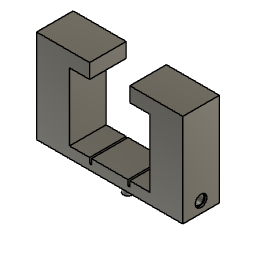
MotorHolder v1 (MostComplicated) (Autodesk Fusion 360 design; units mm, degrees)
Autodesk Fusion 360 part; units mm, degrees
sketch "Sketch1" plane through (0, 0, 0) normal (0, 0, 1) x (1, 0, 0)
  line L0 (25, -9.25) -> (-25, -9.25)
  line L1 (-25, -9.25) -> (-25, 9.25)
  line L2 (-25, 9.25) -> (25, 9.25)
  line L3 (25, 9.25) -> (25, -9.25)
  line L4 (25, -9.25) -> (-25, 9.25) construction
  line L5 (-25, -9.25) -> (25, 9.25) construction
  dimension "d1" = 50
  dimension "d2" = 18.5
  constraint horizontal L0
  constraint perpendicular L0 L1
  constraint parallel L0 L2
  constraint parallel L1 L3
  constraint coincident L4 origin
  constraint coincident L5 origin
  measures "d1" distance of L1.end L2.end
  measures "d2" distance of L0.end L1.end
extrude "Extrude1" add sketch "Sketch1" along normal blind 22 makes body 1
move_body "Move1" bodies 1 to x (0, -1, 0) y (1, 0, 0) z (0, 0, 1) at (9.25, -34.25, 0)
move_body "Move2" bodies 1 to x (1, 0, 0) y (0, 1, 0) z (0, 0, 1) at (0, 34, 0)
sketch "Sketch2" plane through (0, 0, 0) normal (0, 0, 1) x (1, 0, 0)
  line L0 (20, 6) -> (30, 6)
  line L1 (30, 6) -> (30, -8.5)
  line L2 (30, -8.5) -> (20, -8.5)
  line L3 (20, -8.5) -> (20, 6)
  dimension "d5" = 10
  dimension "d6" = 14.5
  constraint horizontal L0
  constraint vertical L1
  constraint horizontal L2
  constraint vertical L3
  measures "d5" distance of L0.start L0.end
  measures "d6" distance of L0.start L2.end
extrude "Extrude2" add sketch "Sketch2" along normal blind 24 separate body makes body 2
move_body "Move3" bodies 1 to x (0, 0, 1) y (0, 1, 0) z (-1, 0, 0) at (11, 0, 0)
move_body "Move4" bodies 2 to x (1, 0, 0) y (0, 1, 0) z (0, 0, 1) at (-9, 0, 0)
move_body "Move5" bodies 2 to x (0, -1, 0) y (1, 0, 0) z (0, 0, 1) at (19.5, 2.5, 0)
move_body "Move6" bodies 2 to x (1, 0, 0) y (0, 1, 0) z (0, 0, 1) at (0, 14, 0)
copy_body "CopyPasteBodies1" bodies 2 makes body 3
move_body "Move7" bodies 3 to x (1, 0, 0) y (0, 1, 0) z (0, 0, 1) at (-37, 0, 0)
sketch "Sketch3" plane through (0, 0, 0) normal (0, 0, 1) x (1, 0, 0)
  line L0 (-6, 4) -> (4, 4)
  line L1 (4, 4) -> (4, -6)
  line L2 (4, -6) -> (-6, -6)
  line L3 (-6, -6) -> (-6, 4)
  dimension "d9" = 10
  dimension "d10" = 10
  constraint horizontal L0
  constraint vertical L1
  constraint horizontal L2
  constraint vertical L3
  measures "d9" distance of L0.start L0.end
  measures "d10" distance of L0.start L2.end
extrude "Extrude3" add sketch "Sketch3" along normal blind 3 separate body makes body 4
move_body "Move8" bodies 4 to x (1, 0, 0) y (0, 1, 0) z (0, 0, 1) at (0, 0, -3)
move_body "Move9" bodies 4 to x (1, 0, 0) y (0, 1, 0) z (0, 0, 1) at (1, 1, 0)
move_body "Move10" bodies 2 3 to x (1, 0, 0) y (0, 1, 0) z (0, 0, 1) at (0, 0, -1.5)
move_body "Move11" bodies 2 to x (1, 0, 0) y (0, 1, 0) z (0, 0, 1) at (-6, 0, 0)
move_body "Move12" bodies 3 to x (1, 0, 0) y (0, 1, 0) z (0, 0, 1) at (6, 0, 0)
move_body "Move13" bodies 3 to x (1, 0, 0) y (0, 1, 0) z (0, 0, 1) at (0.5, 0, 0)
sketch "Sketch4" plane through (0, 0, 18.5) normal (0, 0, 1) x (-1, 0, 0)
  line L0 (-11, 25.25) -> (-11, -24.75)
  line L1 (-11, -24.75) -> (11, -24.75)
  line L2 (11, -24.75) -> (11, 25.25)
  line L3 (11, 25.25) -> (-11, 25.25)
  line L4 (-20, 5) -> (20, 5)
  line L5 (20, 5) -> (20, -5)
  line L6 (20, -5) -> (-20, -5)
  line L7 (-20, -5) -> (-20, 5)
  line L8 (-20, 5) -> (20, -5) construction
  line L9 (20, 5) -> (-20, -5) construction
  dimension "d13" = 40
  dimension "d14" = 10
  constraint horizontal L4
  constraint perpendicular L4 L5
  constraint parallel L4 L6
  constraint parallel L5 L7
  constraint coincident L8 origin
  constraint coincident L9 origin
  measures "d13" distance of L5.end L6.end
  measures "d14" distance of L4.end L5.end
extrude "Extrude4" add sketch "Sketch4" along normal blind 1.5 separate body contours L0 L2 L4 L6 | L0 L4 L6 L7 | L2 L4 L5 L6 makes body 5
move_body "Move14" bodies 5 to x (1, 0, 0) y (0, 1, 0) z (0, 0, 1) at (0, 0, -21.5)
move_body "Move15" bodies 3 to x (1, 0, 0) y (0, 1, 0) z (0, 0, 1) at (-0.5, 0, 0)
move_body "Move16" bodies 2 to x (1, 0, 0) y (0, 1, 0) z (0, 0, 1) at (0.5, 0, 0)
sketch "Sketch5" plane through (0, 0, 0) normal (0, 0, 1) x (1, 0, 0)
  circle A0 centre (0, 0) radius 1.255
  dimension "d17" = 2.51
  constraint coincident A0.centre origin
  measures "d17" diameter of A0
extrude "Extrude5" add sketch "Sketch5" against normal blind 8 bodies 4 5
sketch "Sketch6" plane through (0, 0, -3) normal (0, 0, -1) x (1, 0, 0)
  circle A0 centre (0, 0) radius 1.255
  line L0 (20, 5) -> (-20, 5)
  line L1 (-20, 5) -> (-20, -5)
  line L2 (-20, -5) -> (20, -5)
  line L3 (20, -5) -> (20, 5)
  circle A1 centre (0, 0) radius 1.6
  dimension "d20" = 3.2
  constraint concentric A0 A1
  measures "d20" diameter of A1
extrude "Extrude6" add sketch "Sketch6" along normal blind 0.5 contours A1 bodies 4
sketch "Sketch7" plane through (20, 0, 0) normal (1, 0, 0) x (0, 1, 0)
  line L0 (-4.5, -1.5) -> (5.5, -1.5)
  line L1 (5.5, -1.5) -> (5.5, 22.5)
  line L2 (5.5, 22.5) -> (-4.5, 22.5)
  line L3 (-4.5, 22.5) -> (-4.5, -1.5)
  circle A0 centre (0, 0) radius 1.3
  dimension "d23" = 2.6
  constraint coincident A0.centre origin
  measures "d23" diameter of A0
move_body "Move18" bodies 2 to x (1, 0, 0) y (0, 1, 0) z (0, 0, 1) at (0, -0.5, 0)
move_body "Move19" bodies 3 to x (1, 0, 0) y (0, 1, 0) z (0, 0, 1) at (0, -0.5, 0)
sketch "Sketch9" plane through (20, 0, 0) normal (1, 0, 0) x (0, 1, 0)
  line L0 (-5, -1.5) -> (5, -1.5)
  line L1 (5, -1.5) -> (5, 22.5)
  line L2 (5, 22.5) -> (-5, 22.5)
  line L3 (-5, 22.5) -> (-5, -1.5)
  circle A0 centre (0, 0) radius 1.3
  dimension "d29" = 2.6
  constraint coincident A0.centre origin
  measures "d29" diameter of A0
extrude "Extrude9" cut sketch "Sketch9" against normal blind 8 contours A0 bodies 2
sketch "Sketch10" plane through (20, 0, 0) normal (1, 0, 0) x (0, 1, 0)
  circle A0 centre (0, 0) radius 1.3
  line L0 (-5, -1.5) -> (5, -1.5)
  line L1 (5, -1.5) -> (5, 22.5)
  line L2 (5, 22.5) -> (-5, 22.5)
  line L3 (-5, 22.5) -> (-5, -1.5)
  circle A1 centre (0, 0) radius 1.6
  dimension "d32" = 3.2
  constraint concentric A0 A1
  measures "d32" diameter of A1
combine "Combine1" operation add target body 2 tool bodies 3 4
sketch "Sketch11" plane through (20, 0, 0) normal (1, 0, 0) x (0, 1, 0)
  circle A0 centre (0, 0) radius 1.3
  line L0 (5, -3) -> (5, 22.5)
  line L1 (5, 22.5) -> (-5, 22.5)
  line L2 (-5, 22.5) -> (-5, -3)
  line L3 (-5, -3) -> (5, -3)
  circle A1 centre (0, 0) radius 1.6
  dimension "d35" = 3.2
  constraint concentric A0 A1
  measures "d35" diameter of A1
extrude "Extrude11" cut sketch "Sketch11" against normal blind 0.5 contours A1 bodies 2
sketch "Sketch12" plane through (-20, 0, 0) normal (-1, 0, 0) x (0, -1, 0)
  line L0 (5, -3) -> (5, 22.5)
  line L1 (5, 22.5) -> (-5, 22.5)
  line L2 (-5, 22.5) -> (-5, -3)
  line L3 (-5, -3) -> (5, -3)
  circle A0 centre (0, 0) radius 1.3
  dimension "d38" = 2.6
  constraint coincident A0.centre origin
  measures "d38" diameter of A0
extrude "Extrude12" cut sketch "Sketch12" against normal blind 8 contours A0 bodies 2
sketch "Sketch13" plane through (-20, 0, 0) normal (-1, 0, 0) x (0, -1, 0)
  circle A0 centre (0, 0) radius 1.3
  line L0 (5, -3) -> (5, 22.5)
  line L1 (5, 22.5) -> (-5, 22.5)
  line L2 (-5, 22.5) -> (-5, -3)
  line L3 (-5, -3) -> (5, -3)
  circle A1 centre (0, 0) radius 1.6
  dimension "d41" = 3.2
  constraint coincident A0.centre A1.centre
  measures "d41" diameter of A1
extrude "Extrude13" cut sketch "Sketch13" against normal blind 0.5 contours A1 bodies 2
combine "Combine2" operation cut target body 2 tool bodies 1
extrude "Extrude10" [suppressed]
extrude "Extrude7" [rolled back] along distance -8 taper angle 0
sketch "Sketch8" plane through (20, 0, 0) normal (1, 0, 0) x (0, 1, 0)
  circle A0 centre (0, 0) radius 1.3
  line L0 (-4.5, -1.5) -> (5.5, -1.5)
  line L1 (5.5, -1.5) -> (5.5, 22.5)
  line L2 (5.5, 22.5) -> (-4.5, 22.5)
  line L3 (-4.5, 22.5) -> (-4.5, -1.5)
  circle A1 centre (0, 0) radius 1.6
  dimension "d26" = 3.2
  constraint concentric A0 A1
  measures "d26" diameter of A1
extrude "Extrude8" [rolled back] along distance -0.5 taper angle 0
move_body "Move17" [rolled back]
named bodies: "Body2"
